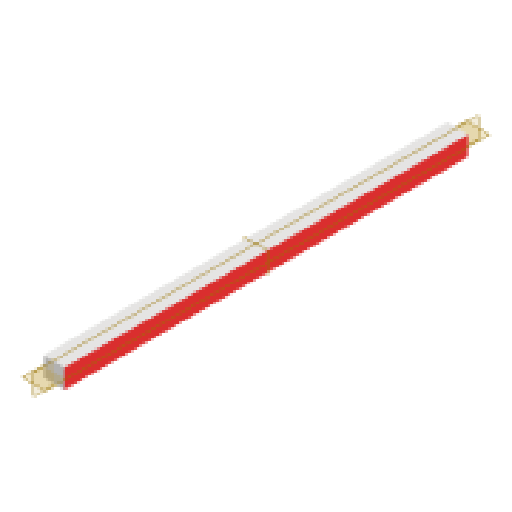
# Autodesk Inventor part: Проставка для боковых фанер
Saved by Autodesk Inventor 2023.2 (Build 272271030, 271C)
## iProperties
Created: 2025-04-24
Part Number: Проставка для боковых фанер
Material: Типовые
Document SubType Name: Modeling
Designer: Коноваленко
Density: 1 g/cm^3
Appearance: По умолчанию
Author: Коноваленко
Autodesk Inventor part; units mm, degrees
sketch "Эскиз1" plane through (0, 0, 0) normal (1, 0, 0) x (0, 1, 0)
  line L0 (-10, -210) -> (10, -210)
  line L1 (10, -210) -> (10, 210)
  line L2 (10, 210) -> (-10, 210)
  line L3 (-10, 210) -> (-10, -210)
  line L4 (-10, -210) -> (10, 210) construction
  line L5 (10, -210) -> (-10, 210) construction
  line L6 (0, 294) -> (0, -294) construction
  line L7 (-14, 0) -> (14, 0) construction
  point P0 (0, 0)
  point P1 (0, 0)
  dimension "d8" = 420
  constraints: 12 end point, 4 midpoint, 2 parallel, 1 horizontal, 1 perpendicular
  measures "d8" distance of L0.end L1.end
extrude "Выдавливание1" add sketch "Эскиз1" along normal mid plane 22
